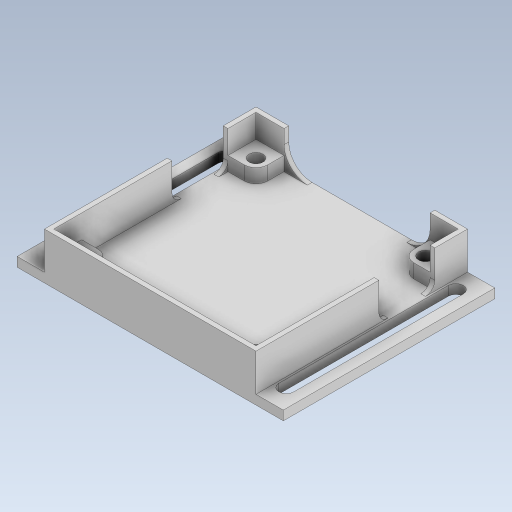
# Autodesk Inventor part: Mounting L298N
Saved by Autodesk Inventor 2023.5 (Build 275446000, 446)
## iProperties
Created: 2025-10-17
Part Number: Mounting L298N
Material: Generic
Document SubType Name: Modeling
Designer: Guntur
Density: 1 g/cm^3
Appearance: Default
Author: Guntur
## iProperties of the stored document Mounting L298N_3DPrint.ipt
Created: 2025-10-27
Part Number: Mounting L298N_3DPrint
Material: Generic
Document SubType Name: Modeling
Designer: Guntur
Density: 1 g/cm^3
Appearance: Default
Author: Guntur
Autodesk Inventor part; units mm, degrees
ref_plane "YZ Plane" through (0, 0, 0) normal (1, 0, 0) x (0, 1, 0)
ref_plane "XZ Plane" through (0, 0, 0) normal (0, 1, 0) x (-1, 0, 0)
ref_plane "XY Plane" through (0, 0, 0) normal (0, 0, 1) x (1, 0, 0)
sketch "Sketch1" plane through (0, 0, 0) normal (0, 1, 0) x (-1, 0, 0)
  line L0 (21.65, 21.65) -> (-21.65, 21.65)
  line L1 (-21.65, 21.65) -> (-21.65, -21.65)
  line L2 (-21.65, -21.65) -> (21.65, -21.65)
  line L3 (21.65, -21.65) -> (21.65, 21.65)
  line L4 (21.65, 21.65) -> (-21.65, -21.65) construction
  line L5 (-21.65, 21.65) -> (21.65, -21.65) construction
  line L6 (22.65, 22.65) -> (-22.65, 22.65)
  line L7 (-22.65, 22.65) -> (-22.65, -22.65)
  line L8 (-22.65, -22.65) -> (22.65, -22.65)
  line L9 (22.65, -22.65) -> (22.65, 22.65)
  line L10 (22.65, 22.65) -> (-22.65, -22.65) construction
  line L11 (-22.65, 22.65) -> (22.65, -22.65) construction
  arc A0 (15.65, 18.15) -> (18.15, 15.65) centre (18.15, 18.15) ccw
  circle A1 centre (18.15, 18.15) radius 1.5
  line L12 (25, 0) -> (-31, 0) construction
  line L13 (0, 28) -> (0, -33) construction
  line L14 (15.65, 18.15) -> (15.65, 21.65)
  line L15 (18.15, 15.65) -> (21.65, 15.65)
  arc A2 (18.15, -15.65) -> (15.65, -18.15) centre (18.15, -18.15) ccw
  circle A3 centre (18.15, -18.15) radius 1.5
  line L16 (15.65, -18.15) -> (15.65, -21.65)
  line L17 (18.15, -15.65) -> (21.65, -15.65)
  arc A4 (-18.15, 15.65) -> (-15.65, 18.15) centre (-18.15, 18.15) ccw
  circle A5 centre (-18.15, 18.15) radius 1.5
  line L18 (-15.65, 18.15) -> (-15.65, 21.65)
  line L19 (-18.15, 15.65) -> (-21.65, 15.65)
  circle A6 centre (-18.15, -18.15) radius 1.5
  line L20 (-18.15, -15.65) -> (-21.65, -15.65)
  line L21 (-15.65, -18.15) -> (-15.65, -21.65)
  arc A7 (-15.65, -18.15) -> (-18.15, -15.65) centre (-18.15, -18.15) ccw
  line L22 (28.5, 22.65) -> (-28.5, 22.65)
  line L23 (-28.5, 22.65) -> (-28.5, -22.65)
  line L24 (-28.5, -22.65) -> (28.5, -22.65)
  line L25 (28.5, -22.65) -> (28.5, 22.65)
  line L26 (28.5, 22.65) -> (-28.5, -22.65) construction
  line L27 (-28.5, 22.65) -> (28.5, -22.65) construction
  line L28 (24.65, 18.15) -> (24.65, -18.15) construction
  line L29 (23.05, 18.15) -> (23.05, -18.15)
  line L30 (26.25, -18.15) -> (26.25, 18.15)
  arc A8 (26.25, 18.15) -> (23.05, 18.15) centre (24.65, 18.15) ccw
  arc A9 (23.05, -18.15) -> (26.25, -18.15) centre (24.65, -18.15) ccw
  line L31 (-24.65, 18.15) -> (-24.65, -18.15) construction
  line L32 (-23.05, 18.15) -> (-23.05, -18.15)
  line L33 (-26.25, -18.15) -> (-26.25, 18.15)
  arc A10 (-23.05, 18.15) -> (-26.25, 18.15) centre (-24.65, 18.15) ccw
  arc A11 (-26.25, -18.15) -> (-23.05, -18.15) centre (-24.65, -18.15) ccw
  point P0 (0, 0)
  point P1 (24.65, 0)
  point P2 (-25, 0)
  point P3 (-24.65, 0)
  point P4 (22.65, 22.65)
  point P5 (22.65, -22.65)
  point P6 (-22.65, -22.65)
  dimension "d0" = 43.3
  dimension "d1" = 43.3
  dimension "d2" = 45.3
  dimension "d3" = 45.3
  dimension "d4" = 5
  dimension "d5" = 3.5
  dimension "d6" = 3.5
  dimension "d7" = 3
  dimension "d14" = 3
  dimension "d15" = 57
  dimension "d16" = 3.2
  dimension "d17" = 2
  dimension "d20" = 45.3
  constraints: 72 end point, 26 symmetric about line, 16 point on circle, 12 centre point, 7 midpoint, 7 parallel, 5 perpendicular, 5 tangent, 4 coincident, 4 horizontal, 2 point on line, 2 vertical, 8 other
  measures "d0" distance of L2.end L1.end
  measures "d1" distance of L1.end L0.end
  measures "d2" distance of L8.end L7.end
  measures "d3" distance of L7.end L6.end
  measures "d4" diameter of A0
  measures "d5" distance from line of L3 A0.centre
  measures "d6" distance from line of L0 A0.centre
  measures "d7" diameter of A1
  measures "d14" diameter of A3
  measures "d15" distance of L24.end L23.end
  measures "d16" diameter of A9
  measures "d17" distance between parallel lines of L9 L28
  measures "d20" distance of L24.end L22.start
extrude "Extrusion1" add sketch "Sketch1" along normal blind 10 contours L9 L8 L7 L6
extrude "Extrusion2" add sketch "Sketch1" along normal blind 2 contours L14 A0 L15 L3 L17 A2 L16 L2 L21 A7 L20 L1 L19 A4 L18 L0
extrude "Extrusion3" add sketch "Sketch1" along normal blind 5 contours L3 L15 A0 L14 L0 | L18 A4 L19 L1 L0 | L3 L2 L16 A2 L17 | L20 A7 L21 L2 L1
extrude "Extrusion4" add sketch "Sketch1" along normal blind 2 contours L22 L25 L24 L9 | L7 L24 L23 L22
sketch "Sketch2" plane through (-21.65, 10, -21.65) normal (0, 0, 1) x (1, 0, 0)
  line L0 (37.3, -8) -> (37.3, -5) projected
  line L1 (0, 0) -> (43.3, 0) projected
  line L2 (32.3, -8) -> (11, -8)
  line L3 (6, -3) -> (6, 0)
  line L4 (6, 0) -> (37.3, 0)
  line L5 (37.3, 0) -> (37.3, -3)
  arc A0 (6, -3) -> (11, -8) centre (11, -3) ccw
  arc A1 (32.3, -8) -> (37.3, -3) centre (32.3, -3) ccw
  point P0 (21.65, -10)
  point P1 (6, -8)
  point P2 (37.3, -5)
  dimension "d23" = 5
  constraints: 8 end point, 5 point on line, 4 point on circle, 4 tangent, 2 centre point, 2 parallel, 1 equal radius, 1 horizontal, 1 perpendicular
  measures "d23" radius of A0
extrude "Extrusion5" cut sketch "Sketch2" against normal blind 2
sketch "Sketch3" plane through (21.65, 10, -21.65) normal (-1, 0, 0) x (0, 0, 1)
  line L0 (6, -8) -> (37.3, -8) projected
  line L1 (8, -8) -> (16, -8)
  line L2 (18, -6) -> (18, 0)
  line L3 (18, 0) -> (6, 0)
  line L4 (6, 0) -> (6, -6)
  arc A0 (6, -6) -> (8, -8) centre (8, -6) ccw
  arc A1 (16, -8) -> (18, -6) centre (16, -6) ccw
  point P0 (21.65, -10)
  dimension "d24" = 2
  constraints: 8 end point, 4 point on circle, 4 tangent, 2 centre point, 2 parallel, 2 point on line, 1 equal radius, 1 horizontal, 1 perpendicular
  measures "d24" radius of A0
extrude "Extrusion6" cut sketch "Sketch3" against normal blind 2
sketch "Sketch4" plane through (-21.65, 10, 21.65) normal (1, 0, 0) x (0, 0, -1)
  line L0 (37.3, -8) -> (37.3, -5) projected
  line L1 (44.3, 0) -> (-1, 0) projected
  line L2 (35.3, -8) -> (27.3, -8)
  line L3 (25.3, -6) -> (25.3, 0)
  line L4 (25.3, 0) -> (37.3, 0)
  line L5 (37.3, 0) -> (37.3, -6)
  arc A0 (25.3, -6) -> (27.3, -8) centre (27.3, -6) ccw
  arc A1 (35.3, -8) -> (37.3, -6) centre (35.3, -6) ccw
  point P0 (21.65, -10)
  dimension "d27" = 12
  dimension "d28" = 2
  constraints: 8 end point, 4 point on circle, 4 tangent, 3 point on line, 2 centre point, 2 parallel, 1 equal radius, 1 horizontal, 1 perpendicular
  measures "d27" distance of L3.end L4.end
  measures "d28" radius of A0
extrude "Extrusion7" cut sketch "Sketch4" against normal blind 2
body "Solid1"
